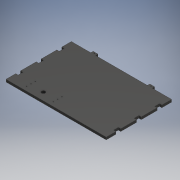
# Autodesk Inventor part: BA02
Saved by Autodesk Inventor 2017 (Build 210142000, 142)
## iProperties
Created: 2019-05-22
Part Number: BA02
Material: Polyethylene, High Density
Document SubType Name: Modeling
Designer: Dell
Density: 0.952 g/cm^3
Appearance: Smooth - Black
Author: Dell
Autodesk Inventor part; units mm, degrees
ref_plane "YZ Plane" through (0, 0, 0) normal (1, 0, 0) x (0, 1, 0)
ref_plane "XZ Plane" through (0, 0, 0) normal (0, 1, 0) x (-1, 0, 0)
ref_plane "XY Plane" through (0, 0, 0) normal (0, 0, 1) x (1, 0, 0)
sketch "Sketch1" plane through (0, 0, 0) normal (0, 0, 1) x (1, 0, 0)
  line L0 (0, 0) -> (525.78, 0)
  line L1 (525.78, 0) -> (525.78, 342.9)
  line L2 (525.78, 342.9) -> (0, 342.9)
  line L3 (0, 342.9) -> (0, 0)
  line L4 (226.36, 66.95) -> (226.36, 21.95) construction
  circle A0 centre (226.36, 66.95) radius 2.3813
  circle A1 centre (226.36, 21.95) radius 2.3813
  circle A2 centre (226.36, 44.45) radius 2.3813
  line L5 (166.36, 29.45) -> (166.36, 49.45) construction
  line L6 (156.36, 66.95) -> (156.36, 21.95) construction
  line L7 (166.36, 49.45) -> (146.36, 49.45) construction
  line L8 (146.36, 29.45) -> (166.36, 29.45) construction
  circle A3 centre (156.36, 39.45) radius 10
  line L9 (226.36, 21.95) -> (86.36, 21.95) construction
  line L10 (86.36, 66.95) -> (226.36, 66.95) construction
  line L11 (86.36, 44.45) -> (226.36, 44.45) construction
  line L12 (146.36, 49.45) -> (146.36, 29.45) construction
  line L13 (0, 0) -> (525.78, 0) construction
  line L14 (525.78, 0) -> (525.78, 88.9)
  line L15 (525.78, 88.9) -> (0, 88.9) construction
  line L16 (0, 88.9) -> (0, 0) construction
  line L17 (86.36, 21.95) -> (86.36, 66.95) construction
  circle A4 centre (86.36, 66.95) radius 2.3812
  circle A5 centre (86.36, 21.95) radius 2.3812
  circle A6 centre (86.36, 44.45) radius 2.3812
  point P0 (166.36, 39.45)
  point P1 (146.36, 39.45)
  point P2 (0, 44.45)
  dimension "d0" = 342.9
  dimension "d1" = 525.78
  dimension "d2" = 45
  dimension "d3" = 140
  dimension "d4" = 4.7625
  dimension "d5" = 4.7625
  dimension "d6" = 4.7625
  dimension "d7" = 4.7625
  dimension "d8" = 4.7625
  dimension "d9" = 4.7625
  dimension "d10" = 60
  dimension "d11" = 7.5
  dimension "d12" = 20
  dimension "d13" = 20
  dimension "d14" = 86.36
  dimension "d15" = 88.9
  constraints: 36 end point, 8 parallel, 7 midpoint, 6 centre point, 5 coincident, 4 perpendicular, 3 horizontal alignment, 2 horizontal, 2 point on line, 2 other
  measures "d0" distance of L2.end L0.start
  measures "d1" distance of L0.start L0.end
  measures "d2" distance of L4.start L4.end
  measures "d3" distance of L17.end L4.start
  measures "d4" diameter of A4
  measures "d5" diameter of A6
  measures "d6" diameter of A5
  measures "d7" diameter of A1
  measures "d8" diameter of A2
  measures "d9" diameter of A0
  measures "d10" distance from line of L11.end L5
  measures "d11" distance between parallel lines of L9 L8
  measures "d12" distance of L5.end L12.start
  measures "d13" distance of L12.start L8.start
  measures "d14" distance between parallel lines of L16 L17
  measures "d15" distance of L15.end L13.start
extrude "Extrusion1" add sketch "Sketch1" along normal blind 12.7
sketch "Sketch2" plane through (0, 0, 12.7) normal (0, 0, 1) x (1, 0, 0)
  line L0 (525.78, 342.9) -> (0, 342.9) projected
  line L1 (101.6, 342.9) -> (127, 342.9)
  line L2 (127, 342.9) -> (127, 355.6)
  line L3 (127, 355.6) -> (101.6, 355.6)
  line L4 (101.6, 355.6) -> (101.6, 342.9)
  line L5 (0, 342.9) -> (0, 0) projected
  line L6 (262.89, 342.9) -> (262.89, 386.8153)
  line L7 (0, 342.9) -> (525.78, 342.9)
  line L8 (424.18, 342.9) -> (398.78, 342.9)
  line L9 (398.78, 342.9) -> (398.78, 355.6)
  line L10 (398.78, 355.6) -> (424.18, 355.6)
  line L11 (424.18, 355.6) -> (424.18, 342.9)
  dimension "d18" = 25.4
  dimension "d19" = 12.7
  dimension "d20" = 101.6
  constraints: 20 end point, 6 symmetric about line, 2 parallel, 2 point on line, 1 horizontal, 1 midpoint, 1 perpendicular, 1 vertical
  measures "d18" distance of L3.end L2.end
  measures "d19" distance of L2.end L1.end
  measures "d20" distance from line of L5 L3.end
extrude "Extrusion2" add sketch "Sketch2" against normal blind 12.7
sketch "Sketch3" plane through (0, 0, 12.7) normal (0, 0, 1) x (1, 0, 0)
  line L0 (101.6, 355.6) -> (101.6, 342.9) projected
  line L1 (127, 355.6) -> (101.6, 355.6) projected
  line L2 (424.18, 355.6) -> (424.18, 342.9) projected
  line L3 (398.78, 355.6) -> (424.18, 355.6) projected
  circle A0 centre (114.3, 349.25) radius 2.25
  circle A1 centre (411.48, 349.25) radius 2.25
  point P0 (0, 0)
  point P1 (114.3, 355.6)
  point P2 (101.6, 349.25)
  point P3 (424.18, 349.25)
  point P4 (411.48, 355.6)
  dimension "d23" = 4.5
  dimension "d24" = 4.5
  constraints: 4 midpoint, 2 centre point, 2 horizontal alignment, 2 vertical alignment
  measures "d23" diameter of A0
  measures "d24" diameter of A1
extrude "Extrusion3" cut sketch "Sketch3" against normal through all
sketch "Sketch4" plane through (0, 0, 12.7) normal (0, 0, 1) x (1, 0, 0)
  line L0 (0, 342.9) -> (0, 0) projected
  line L1 (0, 292.1) -> (12.7, 292.1)
  line L2 (12.7, 292.1) -> (12.7, 266.7)
  line L3 (12.7, 266.7) -> (0, 266.7)
  line L4 (0, 266.7) -> (0, 292.1)
  line L5 (0, 184.15) -> (12.7, 184.15)
  line L6 (12.7, 184.15) -> (12.7, 158.75)
  line L7 (12.7, 158.75) -> (0, 158.75)
  line L8 (0, 158.75) -> (0, 184.15)
  line L9 (0, 50.8) -> (12.7, 50.8)
  line L10 (12.7, 50.8) -> (12.7, 76.2)
  line L11 (12.7, 76.2) -> (0, 76.2)
  line L12 (0, 76.2) -> (0, 50.8)
  line L13 (398.78, 342.9) -> (127, 342.9) projected
  line L14 (262.89, 342.9) -> (262.89, 381.8004)
  line L15 (525.78, 342.9) -> (525.78, 0)
  line L16 (525.78, 292.1) -> (513.08, 292.1)
  line L17 (513.08, 292.1) -> (513.08, 266.7)
  line L18 (513.08, 266.7) -> (525.78, 266.7)
  line L19 (525.78, 266.7) -> (525.78, 292.1)
  line L20 (525.78, 184.15) -> (513.08, 184.15)
  line L21 (513.08, 184.15) -> (513.08, 158.75)
  line L22 (513.08, 158.75) -> (525.78, 158.75)
  line L23 (525.78, 158.75) -> (525.78, 184.15)
  line L24 (525.78, 50.8) -> (513.08, 50.8)
  line L25 (513.08, 50.8) -> (513.08, 76.2)
  line L26 (513.08, 76.2) -> (525.78, 76.2)
  line L27 (525.78, 76.2) -> (525.78, 50.8)
  point P0 (0, 171.45)
  point P1 (525.78, 171.45)
  dimension "d27" = 12.7
  dimension "d28" = 25.4
  dimension "d29" = 12.7
  dimension "d30" = 25.4
  dimension "d31" = 12.7
  dimension "d32" = 25.4
  dimension "d33" = 50.8
  dimension "d34" = 50.8
  constraints: 52 end point, 15 symmetric about line, 6 parallel, 6 point on line, 3 horizontal, 3 midpoint, 3 perpendicular, 1 vertical
  measures "d27" distance of L2.end L3.end
  measures "d28" distance of L1.end L2.end
  measures "d29" distance of L6.end L7.end
  measures "d30" distance of L5.end L6.end
  measures "d31" distance of L11.end L10.end
  measures "d32" distance of L9.end L10.end
  measures "d33" distance from line of L0.start L1
  measures "d34" distance from line of L0.end L9
extrude "Extrusion4" cut sketch "Sketch4" against normal through all
body "Solid1"
